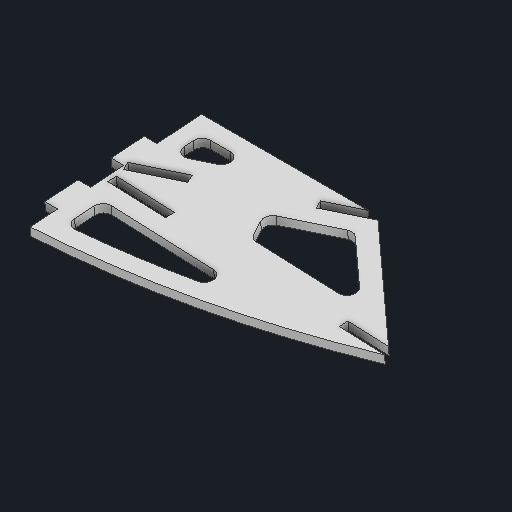
# Autodesk Inventor part: sponson_break
Saved by Autodesk Inventor 2023 (Build 270158030, 158C)
## iProperties
Created: 2022-03-21
Part Number: sponson_break
Material: Generic
Document SubType Name: Modeling
Designer: kardo
Density: 1 g/cm^3
Appearance: Default
Author: kardo
Autodesk Inventor part; units mm, degrees
ref_plane "YZ Plane" through (0, 0, 0) normal (1, 0, 0) x (0, 1, 0)
ref_plane "XZ Plane" through (0, 0, 0) normal (0, 1, 0) x (-1, 0, 0)
ref_plane "XY Plane" through (0, 0, 0) normal (0, 0, 1) x (1, 0, 0)
derived "parameters_frame.ipt"
derived "surface_body.ipt"
sketch "sk_rail_sponson_tunnel" plane through (81.12, 0, 0) normal (1, 0, 0) x (0, 1, 0)
  line L0 (0, 0) -> (111.39, 7.7891)
  line L1 (101.5485, 148.5297) -> (128.7646, -240.679) construction
  spline S0 degree 2 poles (111.39, 7.7891) (176.0348, 12.3096) (237, 36.448) knots 0 0 0 1 1 1
sketch "sk_rail_sponson_bottom" plane through (126.048, 0, 0) normal (0.4037383, -0.0638184, 0.9126459) x (-0.1841621, 0.9714748, 0.1494022)
  line L0 (109.3763, -22.4773) -> (0, 0)
  line L1 (371.255, -76.2945) -> (-489.8119, 100.6585) construction
  line L2 (156.3866, 206.2785) -> (76.3238, -183.3132) construction
  spline S0 degree 2 poles (109.3763, -22.4773) (178.4423, -36.6707) (243.959, 0) knots 0 0 0 1 1 1
  point P0 (23.2133, 112.9576)
sketch "sk_rail_sponson_side" plane through (81.12, 237, 36.448) normal (0.0378267, 0.0348745, -0.9986756) x (0.3011979, -0.9533106, -0.0218819)
  line L0 (248.6073, 0) -> (144.1371, -33.0246)
  spline S0 degree 2 poles (144.1371, -33.0246) (68.7786, -56.8465) (0, 0) knots 0 0 0 1 1 1
  point P0 (202.299, 150.0824)
ref_plane "plane_sponson_break" through (0, 111.39, 7.7891) normal (0, 0.9975641, 0.0697565) x (-1, 0, 0)
sketch "sk_section_sponson_break" plane through (0, 111.39, 7.7891) normal (0, 0.9975641, 0.0697565) x (-1, 0, 0)
  line L0 (-276.1283, -66.2311) -> (62.1846, 83.0679) construction
  line L1 (-81.12, -261.3468) -> (-81.12, 152.2132) construction
  arc A0 (-81.12, 43.0127) -> (-156, 27.1087) centre (-69.8132, -194.4509) ccw construction
  arc A1 (-54.6, 54.2675) -> (-156, 30.9325) centre (-53.2768, -183.4615) ccw construction
  spline S0 degree 2 poles (-54.6, 54.2675) (-107.2974, 54.2675) (-156, 30.9325) knots 0 0 0 1 1 1
  spline S1 degree 2 poles (-156, 27.1087) (-120.096, 41.0753) (-81.12, 43.0127) knots 0 0 0 1 1 1
  point P0 (0, 0)
derived "stencil_frame.ipt"
sketch "sk_joint_locations" plane through (81.12, 0, 0) normal (1, 0, 0) x (0, 1, 0)
  line L0 (0, 0) -> (111.39, 7.7891) construction
  line L1 (30.81, 28.832) -> (94.8, 28.832) construction
  arc A0 (30.81, 28.832) -> (9.48, 28.4869) centre (30.81, -630.4631) ccw construction
  line L2 (-254.1001, 19.9549) -> (9.48, 28.4869) construction
  line L3 (-363, 18.496) -> (-275.8801, 19.4795) construction
  arc A1 (-275.8801, 19.4795) -> (-254.1001, 19.9549) centre (-287.5515, 1053.3708) ccw construction
  line L4 (1.436, 1580.2049) -> (243.9436, -1887.8151) construction
  line L5 (-242.0001, 1541.8302) -> (-242.0001, -1877.3857) construction
  line L6 (-120.9999, 1541.8302) -> (-120.9999, -1877.3857) construction
  line L7 (-363, 1541.8302) -> (-363, -1877.3857) construction
  line L8 (0, 1541.8302) -> (0, -1877.3857) construction
  line L9 (445.406, 43.7257) -> (-613.1443, 6.7603) construction
  line L10 (-676.709, -27.4448) -> (497.0858, 54.635) construction
  line L11 (178.2183, 30.3929) -> (177.9391, 38.388) construction
  line L12 (185.9231, 36.8959) -> (186.4825, 28.8959) construction
  line L13 (0, 6.528) -> (111.1168, 11.6964) construction
  line L14 (-242.0001, 45.8501) -> (-242.0001, 20.3465) construction
  line L15 (-363, 37.4293) -> (-363, 18.496) construction
  line L16 (-120.9999, 51.0063) -> (-120.9999, 24.2633) construction
  line L17 (0, 52.89) -> (0, 28.18) construction
  line L18 (108.3896, 50.6971) -> (108.935, 42.897) construction
  line L19 (109.4805, 35.0968) -> (108.935, 42.897) construction
  line L20 (109.4805, 35.0968) -> (110.0259, 27.2967) construction
  line L21 (110.0259, 27.2967) -> (110.5713, 19.4965) construction
  line L22 (110.5713, 19.4965) -> (111.1168, 11.6964) construction
  line L23 (0, 6.528) -> (0, 0) construction
  spline S0 degree 4 poles (-363, 37.4293) (-272.3626, 45.1427) (-181.5879, 49.7528) (-90.8131, 52.89) (0, 52.89) knots 0 0 0 0 0 1 1 1 1 1
  spline S1 degree 3 poles (0, 52.89) (86.3106, 52.89) (181.3207, 49.5034) (237, 36.448) knots 0 0 0 0 1 1 1 1
  spline S2 degree 2 poles (111.39, 7.7891) (176.0348, 12.3096) (237, 36.448) knots 0 0 0 1 1 1
  line L24 (94.8, 37.536) -> (94.8, 28.832) construction
  line L25 (94.8, 35.548) -> (94.8, 30.82) construction
  point P0 (1.436, 1580.2049)
  point P1 (243.9436, -1887.8151)
  point P2 (178.0787, 34.3904)
  point P3 (186.2028, 32.8959)
  point P4 (134.9575, 11.3411)
  point P5 (-363, 27.9627)
  point P6 (-242.0001, 33.0983)
  point P7 (-120.9999, 37.6348)
  point P8 (0, 40.535)
  point P9 (94.8, 33.184)
sketch "sk_spanner_joints_locations" plane through (0, 111.39, 7.7891) normal (0, 0.9975641, 0.0697565) x (-1, 0, 0)
  line L0 (280.557, 10.5733) -> (-334.5102, 33.8701) construction
  line L1 (-953.5208, -365.1675) -> (735.9219, 380.3912) construction
  line L2 (-85.1788, 24.4262) -> (-84.0523, 18.5329) construction
  line L3 (-85.1788, 24.4262) -> (-71.8427, 23.9211) construction
  line L4 (-84.0523, 18.5329) -> (-71.8427, 23.9211) construction
  point P0 (0, 0)
  point P1 (-126.048, 0)
  point P2 (-156, 27.1087)
  point P3 (-141.8358, 26.5722)
  point P4 (-99.343, 24.9627)
  point P5 (-94.5512, 13.8997)
  point P6 (-115.5491, 4.6332)
sketch "sk_sponson_break_base" plane through (0, 111.39, 7.7891) normal (0, 0.9975641, 0.0697565) x (-1, 0, 0)
  spline S0 degree 2 poles (-156, 27.1087) (-120.096, 41.0753) (-81.12, 43.0127) knots 0 0 0 1 1 1 construction
  line L0 (-156, 27.1087) -> (-126.048, 0) construction
  line L1 (-126.048, 0) -> (-81.12, 0) construction
  line L2 (-81.12, 35.1935) -> (-81.12, 27.3744)
  line L3 (-81.12, 27.3744) -> (-84.12, 27.3744)
  line L4 (-81.12, 35.1935) -> (-84.12, 35.1935)
  line L5 (-84.12, 35.1935) -> (-84.12, 41.6432)
  line L6 (-84.12, 27.3744) -> (-84.12, 19.5552)
  line L7 (-84.12, 19.5552) -> (-81.12, 19.5552)
  line L8 (-81.12, 19.5552) -> (-81.12, 11.736)
  line L9 (-81.12, 11.736) -> (-84.12, 11.736)
  line L10 (-84.12, 11.736) -> (-84.12, 1.2)
  line L11 (-153.7477, 26.6887) -> (-125.5856, 1.2)
  line L12 (-125.5856, 1.2) -> (-84.12, 1.2)
  spline S1 degree 5 poles (-84.12, 41.6432) (-98.39, 40.7571) (-112.5959, 38.8404) (-126.6352, 35.8392) (-140.3812, 31.7634) (-153.7477, 26.6887) knots 0 0 0 0 0 0 1 1 1 1 1 1
  point P0 (0, 0)
  point P1 (-156, 27.1087)
  dimension "d4" = 1.2
  dimension "d3" = 3
  constraints: 26 end point, 6 parallel, 4 perpendicular, 1 vertical, 4 other
  measures "d3" distance from line of L7.end L6
extrude "thicken" add sketch "sk_sponson_break_base" against normal blind 2
sketch "sk_spanner_joints" plane through (0, 111.39, 7.7891) normal (0, 0.9975641, 0.0697565) x (-1, 0, 0)
  line L0 (-156, 27.1087) -> (-141.8358, 26.5722)
  line L1 (-141.8358, 26.5722) -> (-141.9115, 24.5736)
  line L2 (-141.9115, 24.5736) -> (-156.0757, 25.1101)
  line L3 (-156.0757, 25.1101) -> (-156, 27.1087)
  line L4 (-99.343, 24.9627) -> (-99.4187, 22.9641)
  line L5 (-99.4187, 22.9641) -> (-85.2545, 22.4276)
  line L6 (-85.2545, 22.4276) -> (-85.1788, 24.4262)
  line L7 (-99.343, 24.9627) -> (-85.1788, 24.4262)
  line L8 (-94.5512, 13.8997) -> (-95.3587, 15.7294)
  line L9 (-95.3587, 15.7294) -> (-84.8598, 20.3626)
  line L10 (-84.8598, 20.3626) -> (-84.0523, 18.5329)
  line L11 (-84.0523, 18.5329) -> (-94.5512, 13.8997)
  line L12 (-126.048, 0) -> (-115.5491, 4.6332)
  line L13 (-115.5491, 4.6332) -> (-116.3566, 6.463)
  line L14 (-116.3566, 6.463) -> (-126.8555, 1.8297)
  line L15 (-126.8555, 1.8297) -> (-126.048, 0)
  point P0 (0, 0)
  dimension "d7" = 2
  constraints: 32 end point, 8 perpendicular, 7 equal length
  measures "d7" distance of L2.end L0.start
extrude "cut_spanner_joints" cut sketch "sk_spanner_joints" along normal through all both and the other way through all
sketch "sk_cut_weight" plane through (0, 111.39, 7.7891) normal (0, 0.9975641, 0.0697565) x (-1, 0, 0)
  spline S0 degree 3 poles (-84.12, 41.6432) (-88.1375, 41.3938) (-95.1243, 40.7876) (-103.0218, 39.7558) (-108.9077, 38.8366) (-112.8129, 38.1512) (-117.6711, 37.2035) (-121.5391, 36.3728) (-126.3508, 35.2435) (-130.1817, 34.2674) (-134.947, 32.9564) (-138.7407, 31.8349) (-143.4598, 30.3422) (-148.1557, 28.7587) (-151.8878, 27.3949) (-153.7477, 26.6887) knots 0.025406 0.025406 0.025406 0.025406 0.181255 0.298142 0.337104 0.415028 0.45399 0.531915 0.570877 0.648802 0.687764 0.765688 0.80465 0.882575 0.960499 0.960499 0.960499 0.960499 construction
  line L0 (-153.7477, 26.6887) -> (-125.5856, 1.2) construction
  line L1 (-125.5856, 1.2) -> (-84.12, 1.2) construction
  line L2 (-85.1788, 24.4262) -> (-156, 27.1087) construction
  line L3 (-84.0523, 18.5329) -> (-126.048, 0) construction
  line L4 (-80.5816, 22.2506) -> (-151.8257, 24.9491) construction
  line L5 (-80.5816, 22.2506) -> (-126.4696, 2.0001) construction
  line L6 (-84.12, 41.6432) -> (-84.12, 1.2) construction
  line L7 (-88.12, 37.3497) -> (-88.12, 28.5405)
  line L8 (-88.12, 28.5405) -> (-130.1141, 30.1311)
  line L9 (-104.8528, 1.2) -> (-116.2036, 23.5999) construction
  line L10 (-140.9885, 20.5358) -> (-114.1355, 19.5187)
  line L11 (-110.9454, 13.2231) -> (-125.7099, 6.7075)
  line L12 (-125.7099, 6.7075) -> (-140.9885, 20.5358)
  line L13 (-114.1355, 19.5187) -> (-110.9454, 13.2231)
  line L14 (-88.12, 12.3656) -> (-104.3573, 5.2)
  line L15 (-104.3573, 5.2) -> (-88.12, 5.2)
  line L16 (-88.12, 5.2) -> (-88.12, 12.3656)
  spline S1 degree 4 poles (-88.12, 37.3496) (-98.7534, 36.5014) (-109.3384, 35.0257) (-119.8113, 32.8963) (-130.1141, 30.131) knots 0 0 0 0 0 1 1 1 1 1
  point P0 (0, 0)
  dimension "d12" = 4
  dimension "d10" = 2
  dimension "d11" = 2
  dimension "d13" = 4
  dimension "d14" = 4
  dimension "d15" = 4
  dimension "d16" = 4
  dimension "d17" = 4
  dimension "d18" = 4
  dimension "d19" = 4
  dimension "d20" = 4
  constraints: 30 end point, 10 parallel, 4 point on line, 2 midpoint, 3 other
  measures "d10" distance between parallel lines of L2 L4
  measures "d11" distance between parallel lines of L3 L5
  measures "d13" distance between parallel lines of L2 L8
  measures "d14" distance between parallel lines of L6 L7
  measures "d15" distance between parallel lines of L0 L12
  measures "d16" distance between parallel lines of L4 L10
  measures "d17" distance between parallel lines of L5 L11
  measures "d18" distance between parallel lines of L1 L15
  measures "d19" distance between parallel lines of L6 L16
  measures "d20" distance between parallel lines of L3 L14
extrude "cut_weight" cut sketch "sk_cut_weight" along normal through all both and the other way through all
fillet "Fillet1" radius 2 10 edges at (104.3573, 110.0297, 12.9067) (88.12, 109.5299, 20.0549) (88.12, 110.0297, 12.9067) (125.7099, 109.9245, 14.4106) (110.9454, 109.47, 20.9103) (88.12, 108.4016, 36.1903) (114.1355, 109.0309, 27.1905) (140.9885, 108.9599, 28.2052) (130.1141, 108.2906, 37.777) (88.12, 107.7871, 44.9781)
equation "\"d4\" = shell_thickness"
equation "\"d3\" = stringer_thickness"
equation "\"d5\" = bulkhead_thickness"
equation "\"d7\" = bulkhead_thickness"
equation "\"d12\" = bulkhead_inset"
equation "\"d10\" = bulkhead_thickness"
equation "\"d11\" = bulkhead_thickness"
equation "\"d13\" = bulkhead_inset"
equation "\"d14\" = bulkhead_inset"
equation "\"d15\" = bulkhead_inset"
equation "\"d16\" = bulkhead_inset"
equation "\"d17\" = bulkhead_inset"
equation "\"d18\" = bulkhead_inset"
equation "\"d19\" = bulkhead_inset"
equation "\"d20\" = bulkhead_inset"
equation "\"d23\" = 0.5 * bulkhead_inset"
equation "\"shell_thickness\" = 1.2"
equation "\"stringer_thickness\" = 3"
equation "\"bulkhead_thickness\" = 2"
equation "\"bulkhead_inset\" = 4"
body "Solid1"
